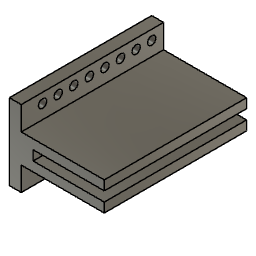
Sensor braket til Kevin v1 (Autodesk Fusion 360 design; units mm, degrees)
Autodesk Fusion 360 part; units mm, degrees
sketch "Sketch1" plane through (0, 0, 0) normal (0, 1, 0) x (1, 0, 0)
  line L0 (37.303, -16.4637) -> (7.303, -16.4637)
  line L1 (-2.697, -16.4637) -> (-2.697, -12.4637)
  line L2 (2.303, -12.4637) -> (37.303, -12.4637)
  line L3 (37.303, -12.4637) -> (37.303, -16.4637)
  line L4 (37.303, -18.5137) -> (-5.6588, -18.5137) construction
  line L5 (2.303, -24.5637) -> (37.303, -24.5637)
  line L6 (-2.697, -20.5637) -> (-2.697, -24.5637)
  line L7 (37.303, -20.5637) -> (7.303, -20.5637)
  line L8 (37.303, -24.5637) -> (37.303, -20.5637)
  line L9 (-2.697, -16.4637) -> (-2.697, -20.5637)
  line L10 (7.303, -16.4637) -> (7.303, -20.5637)
  line L11 (2.303, -12.4637) -> (2.303, -2.4637)
  line L12 (2.303, -2.4637) -> (-2.697, -2.4637)
  line L13 (-2.697, -2.4637) -> (-2.697, -12.4637)
  line L14 (-2.697, -34.5637) -> (-2.697, -24.5637)
  line L15 (2.303, -34.5637) -> (-2.697, -34.5637)
  line L16 (2.303, -24.5637) -> (2.303, -34.5637)
  dimension "d4" = 4
  dimension "d5" = 10
  dimension "d6" = 5
  dimension "d7" = 10
  constraint horizontal L0
  constraint vertical L1
  constraint horizontal L2
  constraint vertical L3
  constraint symmetric L0.start L4 L7.start
  constraint symmetric L1.start L4 L6.start
  constraint symmetric L1.end L4 L6.end
  constraint symmetric L2.end L4 L5.end
  constraint perpendicular L7 L9
  constraint perpendicular L7 L10
  constraint vertical L11
  constraint horizontal L12
  constraint vertical L13
  constraint symmetric L4 L2.start L5.start
  constraint symmetric L4 L11.end L15.start
  constraint symmetric L4 L12.end L14.start
  measures "d4" distance of L0.start L2.end
  measures "d5" distance of L9 L10
  measures "d6" distance of L1.end L2.start
  measures "d7" distance of L1.end L12.end
extrude "Extrude1" add sketch "Sketch1" along normal blind 60
sketch "Sketch2" plane through (-2.697, 0, 0) normal (-1, 0, 0) x (0, -1, 0)
  line L0 (0, 2.4637) -> (0, 34.5637)
  line L1 (0, 34.5637) -> (-60, 34.5637)
  line L2 (-60, 34.5637) -> (-60, 2.4637)
  line L3 (-60, 2.4637) -> (0, 2.4637)
  circle A0 centre (-55, 7.4637) radius 1.75
  circle A1 centre (-48.4286, 7.4637) radius 1.75
  circle A2 centre (-41.8571, 7.4637) radius 1.75
  circle A3 centre (-35.2857, 7.4637) radius 1.75
  circle A4 centre (-28.7143, 7.4637) radius 1.75
  circle A5 centre (-22.1429, 7.4637) radius 1.75
  circle A6 centre (-15.5714, 7.4637) radius 1.75
  circle A7 centre (-9, 7.4637) radius 1.75
  circle A8 centre (-55, 30.4637) radius 1.75
  circle A9 centre (-48.4286, 30.4637) radius 1.75
  circle A10 centre (-41.8571, 30.4637) radius 1.75
  circle A11 centre (-35.2857, 30.4637) radius 1.75
  circle A12 centre (-28.7143, 30.4637) radius 1.75
  circle A13 centre (-22.1429, 30.4637) radius 1.75
  circle A14 centre (-15.5714, 30.4637) radius 1.75
  circle A15 centre (-9, 30.4637) radius 1.75
  dimension "d10" = 3.5
  dimension "d11" = 5
  dimension "d12" = 5
  dimension "d15" = 46
  dimension "d16" = 0
  dimension "d17" = 3.5
  dimension "d18" = 28
  dimension "d21" = 46
  dimension "d22" = 0
  measures "d10" diameter of A0
  measures "d11" distance of L3 A0.centre
  measures "d12" distance of L2 A0.centre
  measures "d17" diameter of A8
  measures "d18" distance of L3 A8.centre
extrude "Extrude2" cut sketch "Sketch2" against normal blind 11 contours A0 | A1 | A2 | A3 | A4 | A5 | A6 | A7 | A8 | A9 | A10 | A11 | A12 | A13 | A14 | A15
